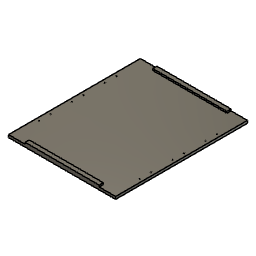
Chasis Sumo v2 (Autodesk Fusion 360 design; units mm, degrees)
Autodesk Fusion 360 part; units mm, degrees
sketch "Esquisse1" plane through (0, 0, 0) normal (0, 1, 0) x (1, 0, 0)
  line L0 (0, 0) -> (130, 0)
  line L1 (130, 0) -> (130, -160)
  line L2 (130, -160) -> (0, -160)
  line L3 (0, -160) -> (0, 0)
  line L4 (130, -87.001) -> (126, -87.001)
  circle A0 centre (126, -87.001) radius 0.5
  circle A1 centre (126.0123, -72.9994) radius 0.5
  line L5 (130.0123, -72.9994) -> (126.0123, -72.9994)
  line L6 (120, 0) -> (120, -80)
  line L7 (120, -80) -> (120, -73)
  line L8 (120, -80) -> (120, -87)
  line L9 (120, 0) -> (120, -40)
  line L10 (120, -40) -> (120, -60)
  line L11 (120, -60) -> (125, -60)
  line L12 (130.0123, -47.0006) -> (126.0123, -47.0006)
  circle A2 centre (126.0123, -47.0006) radius 0.5
  circle A3 centre (126, -32.999) radius 0.5
  line L13 (130, -32.999) -> (126, -32.999)
  line L14 (120, -80) -> (108.5, -80)
  line L15 (130, -127.001) -> (126, -127.001)
  circle A4 centre (126, -127.001) radius 0.5
  line L16 (130.0123, -112.9994) -> (126.0123, -112.9994)
  circle A5 centre (126.0123, -112.9994) radius 0.5
  line L17 (65, 0) -> (65, -160)
  circle A6 centre (4, -32.999) radius 0.5
  line L18 (0, -32.999) -> (4, -32.999)
  circle A7 centre (3.9877, -47.0006) radius 0.5
  line L19 (-0.0123, -47.0006) -> (3.9877, -47.0006)
  line L20 (-0.0123, -72.9994) -> (3.9877, -72.9994)
  circle A8 centre (3.9877, -72.9994) radius 0.5
  line L21 (0, -87.001) -> (4, -87.001)
  circle A9 centre (4, -87.001) radius 0.5
  line L22 (-0.0123, -112.9994) -> (3.9877, -112.9994)
  circle A10 centre (3.9877, -112.9994) radius 0.5
  line L23 (0, -127.001) -> (4, -127.001)
  circle A11 centre (4, -127.001) radius 0.5
  dimension "d1" = 130
  dimension "d2" = 160
  dimension "d5" = 4
  dimension "d6" = 1
  dimension "d16" = 80
  dimension "d17" = 7
  dimension "d18" = 7
  dimension "d19" = 40
  dimension "d20" = 20
  constraint horizontal L0
  constraint vertical L1
  constraint horizontal L2
  constraint coincident L0.start L3.end
  constraint coincident L1 L4.start
  constraint perpendicular L1 L4
  constraint coincident L4.end A0.centre
  constraint coincident L0 L6.start
  constraint perpendicular L0 L6
  constraint parallel L6 L7
  constraint coincident A1.centre L5.end
  constraint parallel L7 L8
  constraint perpendicular L0 L9
  constraint parallel L6 L10
  constraint perpendicular L6 L11
  constraint symmetric L4.start L11 L13.start
  constraint symmetric L4.end L11 A3.centre
  constraint symmetric A0 L11 A3
  constraint symmetric A1 L11 A2
  constraint symmetric L5.start L11 L12.start
  constraint symmetric A1.centre L11 L12.end
  constraint perpendicular L6 L14
  constraint symmetric L12.start L14 L16.start
  constraint symmetric L12.end L14 L16.end
  constraint symmetric A2 L14 A5
  constraint symmetric A3 L14 A4
  constraint symmetric L13.start L14 L15.start
  constraint symmetric A3.centre L14 L15.end
  constraint midpoint L0 L17.start
  constraint midpoint L2 L17.end
  constraint perpendicular L2 L17
  constraint symmetric L4.start L17 L21.start
  constraint symmetric L4.end L17 L21.end
  constraint symmetric A0 L17 A9
  constraint symmetric A1 L17 A8
  constraint symmetric L5.start L17 L20.start
  constraint symmetric A1.centre L17 L20.end
  constraint symmetric L12.start L17 L19.start
  constraint symmetric L12.end L17 A7.centre
  constraint symmetric A2 L17 A7
  constraint symmetric A3 L17 A6
  constraint symmetric L13.start L17 L18.start
  constraint symmetric A3.centre L17 A6.centre
  constraint symmetric L15.start L17 L23.start
  constraint symmetric L15.end L17 L23.end
  constraint symmetric A4 L17 A11
  constraint symmetric L16.start L17 L22.start
  constraint symmetric L16.end L17 L22.end
  constraint symmetric A5 L17 A10
  measures "d1" distance of L0.start L0.end
  measures "d2" distance of L0.start L2.end
  measures "d5" distance of L4.start L4.end
  measures "d6" diameter of A0
  measures "d16" distance of L6.start L6.end
  measures "d17" distance of L6.end L7.end
  measures "d18" distance of L6.end L8.end
  measures "d19" distance of L6.start L9.end
  measures "d20" distance of L9.end L10.end
extrude "Extrusion1" add sketch "Esquisse1" along normal blind 3
sketch "Esquisse2" plane through (0, 3, 0) normal (0, 1, 0) x (-1, 0, 0)
  circle A0 centre (-126, 87.001) radius 0.5
  circle A1 centre (-126.0123, 72.9994) radius 0.5
  line L0 (0, 160) -> (-130, 160)
  line L1 (-130, 160) -> (-130, 0)
  line L2 (-130, 0) -> (0, 0)
  line L3 (0, 0) -> (0, 160)
  line L4 (-20, 0) -> (-110, 0)
  line L5 (-110, 0) -> (-110, 5)
  line L6 (-110, 5) -> (-20, 5)
  line L7 (-20, 5) -> (-20, 0)
  circle A2 centre (-4, 127.001) radius 0.5
  circle A3 centre (-3.9877, 112.9994) radius 0.5
  circle A4 centre (-4, 87.001) radius 0.5
  circle A5 centre (-4, 32.999) radius 0.5
  circle A6 centre (-3.9877, 47.0006) radius 0.5
  circle A7 centre (-126, 127.001) radius 0.5
  circle A8 centre (-126.0123, 112.9994) radius 0.5
  circle A9 centre (-126.0123, 47.0006) radius 0.5
  circle A10 centre (-126, 32.999) radius 0.5
  circle A11 centre (-3.9877, 72.9994) radius 0.5
  line L8 (0, 80) -> (-130, 80)
  line L9 (-110, 155) -> (-20, 155)
  line L10 (-20, 155) -> (-20, 160)
  line L11 (-20, 160) -> (-110, 160)
  line L12 (-110, 160) -> (-110, 155)
  constraint horizontal L4
  constraint vertical L5
  constraint horizontal L6
  constraint vertical L7
  constraint coincident L2 L4.start
  constraint midpoint L3 L8.start
  constraint midpoint L1 L8.end
  constraint symmetric L4.start L8 L10.end
  constraint symmetric L4.end L8 L11.end
  constraint symmetric L5.end L8 L9.start
  constraint symmetric L6.end L8 L9.end
extrude "Extrusion2" add sketch "Esquisse2" along normal blind 2 contours L0 L9 L10 L11 L12 | L2 L4 L5 L6 L7
